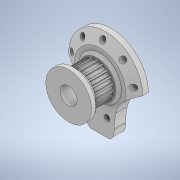
# Autodesk Inventor part: bone_upper_wheel_1
Saved by Autodesk Inventor 2020 (Build 240168000, 168)
## iProperties
Created: 2019-05-05
Part Number: bone_upper_wheel_1
Material: Generic
Document SubType Name: Modeling
Designer: psrob
Density: 1 g/cm^3
Appearance: Default
Author: psrob
Autodesk Inventor part; units mm, degrees
ref_plane "YZ Plane" through (0, 0, 0) normal (1, 0, 0) x (0, 1, 0)
ref_plane "XZ Plane" through (0, 0, 0) normal (0, 1, 0) x (-1, 0, 0)
ref_plane "XY Plane" through (0, 0, 0) normal (0, 0, 1) x (1, 0, 0)
sketch "Sketch1" plane through (0, 0, 0) normal (0, 0, 1) x (1, 0, 0)
  circle A0 centre (0, 18.5) radius 1 projected
  circle A1 centre (7.0707, 15.9265) radius 1 projected
  circle A2 centre (-7.0707, 15.9265) radius 1 projected
  circle A3 centre (10.8329, 9.4101) radius 1 projected
  circle A4 centre (-10.8329, 9.4101) radius 1 projected
  circle A5 centre (0, 7.5) radius 5 projected
  ellipse E0 centre (3, -5.8944) end of major axis (3, -9.5) minor radius 2 (3, -9.5) -> (5, -5.8944) ccw projected
  line L0 (5, -5.8944) -> (5, -5.5) projected
  arc A6 (5.5977, -0.4461) -> (5, -5.5) centre (26.6667, -5.5) ccw projected
  arc A7 (10.155, 5.7831) -> (5.5977, -0.4461) centre (15.3218, -2.7787) ccw projected
  line L1 (10.155, 5.7831) -> (13, 7.5) projected
  arc A8 (13, 7.5) -> (-13, 7.5) centre (0, 7.5) ccw projected
  line L2 (-13, 7.5) -> (-10.155, 5.7831) projected
  arc A9 (-5.5977, -0.4461) -> (-10.155, 5.7831) centre (-15.3218, -2.7787) ccw projected
  arc A10 (-5, -5.5) -> (-5.5977, -0.4461) centre (-26.6667, -5.5) ccw projected
  line L3 (-5, -5.5) -> (-5, -5.8944) projected
  ellipse E1 centre (-3, -5.8944) end of major axis (-3, -9.5) minor radius 2 (-5, -5.8944) -> (-3, -9.5) ccw projected
  line L4 (-3, -9.5) -> (3, -9.5) projected
  circle A11 centre (-2.5, -3.5) radius 1 projected
  circle A12 centre (2.5, -3.5) radius 1 projected
  point P0 (0, 0)
  constraints: 2 other
extrude "Extrusion1" add sketch "Sketch1" along normal blind 4 contours A5 | L4 E1 L3 A10 A9 L2 A8 L1 A7 A6 L0 E0
sketch "Sketch2" plane through (0, 0, 4) normal (0, 0, 1) x (1, 0, 0)
  circle A0 centre (0, 7.5) radius 3 projected
  circle A1 centre (0, 7.5) radius 3
  point P0 (0, 0)
  dimension "d2" = 6
  constraints: 1 centre point, 1 coincident
  measures "d2" diameter of A1
extrude "Extrusion2" cut sketch "Sketch2" against normal blind 3
sketch "Sketch3" plane through (0, 0, 4) normal (0, 0, 1) x (1, 0, 0)
  circle A0 centre (0, 7.5) radius 2.5 projected
  arc A1 (3.5741, 2.5417) -> (3.6111, 2.7467) centre (3.4864, 2.6633) ccw projected
  arc A2 (3.4957, 2.9808) -> (3.6111, 2.7467) centre (4.4426, 3.3021) ccw projected
  arc A3 (4.2392, 3.6696) -> (3.4957, 2.9808) centre (4.0212, 3.1591) ccw projected
  arc A4 (4.4638, 3.5366) -> (4.2392, 3.6696) centre (3.8465, 2.7499) ccw projected
  arc A5 (4.4638, 3.5366) -> (4.671, 3.5579) centre (4.5564, 3.6546) ccw projected
  arc A6 (4.671, 3.5579) -> (4.9313, 3.8888) centre (0, 7.5) ccw projected
  arc A7 (4.9313, 3.8888) -> (4.9032, 4.0952) centre (4.8103, 3.9774) ccw projected
  arc A8 (4.7211, 4.2822) -> (4.9032, 4.0952) centre (5.5224, 4.8804) ccw projected
  arc A9 (5.2154, 5.167) -> (4.7211, 4.2822) centre (5.1658, 4.6142) ccw projected
  arc A10 (5.4701, 5.11) -> (5.2154, 5.167) centre (5.1261, 4.171) ccw projected
  arc A11 (5.4701, 5.11) -> (5.6606, 5.1942) centre (5.5217, 5.2508) ccw projected
  arc A12 (5.6606, 5.1942) -> (5.8059, 5.5894) centre (0, 7.5) ccw projected
  arc A13 (5.8059, 5.5894) -> (5.7154, 5.777) centre (5.6634, 5.6363) ccw projected
  arc A14 (5.4844, 5.8986) -> (5.7154, 5.777) centre (6.0616, 6.7152) ccw projected
  arc A15 (5.681, 6.8928) -> (5.4844, 5.8986) centre (5.8047, 6.3518) ccw projected
  arc A16 (5.9409, 6.9173) -> (5.681, 6.8928) centre (5.9039, 5.918) ccw projected
  arc A17 (5.9409, 6.9173) -> (6.0961, 7.0563) centre (5.9465, 7.0672) ccw projected
  arc A18 (6.0961, 7.0563) -> (6.1122, 7.477) centre (0, 7.5) ccw projected
  arc A19 (6.1122, 7.477) -> (5.9681, 7.6275) centre (5.9622, 7.4776) ccw projected
  arc A20 (5.7108, 7.6717) -> (5.9681, 7.6275) centre (6.0075, 8.6267) ccw projected
  arc A21 (5.5906, 8.6781) -> (5.7108, 7.6717) centre (5.8754, 8.2017) ccw projected
  arc A22 (5.8302, 8.7817) -> (5.5906, 8.6781) centre (6.1038, 7.8198) ccw projected
  arc A23 (5.8302, 8.7817) -> (5.9348, 8.9618) centre (5.7892, 8.9259) ccw projected
  arc A24 (5.9348, 8.9618) -> (5.8201, 9.3669) centre (0, 7.5) ccw projected
  arc A25 (5.8201, 9.3669) -> (5.6366, 9.4655) centre (5.6773, 9.3211) ccw projected
  arc A26 (5.3782, 9.4281) -> (5.6366, 9.4655) centre (5.3653, 10.428) ccw projected
  arc A27 (4.9529, 10.348) -> (5.3782, 9.4281) centre (5.371, 9.983) ccw projected
  arc A28 (5.1488, 10.5206) -> (4.9529, 10.348) centre (5.7063, 9.6904) ccw projected
  arc A29 (5.1488, 10.5206) -> (5.1926, 10.7242) centre (5.0652, 10.6451) ccw projected
  arc A30 (5.1926, 10.7242) -> (4.9583, 11.0741) centre (0, 7.5) ccw projected
  arc A31 (4.9583, 11.0741) -> (4.7533, 11.1111) centre (4.8367, 10.9864) ccw projected
  arc A32 (4.5192, 10.9957) -> (4.7533, 11.1111) centre (4.1979, 11.9426) ccw projected
  arc A33 (3.8304, 11.7392) -> (4.5192, 10.9957) centre (4.3409, 11.5212) ccw projected
  arc A34 (3.9634, 11.9638) -> (3.8304, 11.7392) centre (4.7501, 11.3465) ccw projected
  arc A35 (3.9634, 11.9638) -> (3.9421, 12.171) centre (3.8454, 12.0564) ccw projected
  arc A36 (3.9421, 12.171) -> (3.6112, 12.4313) centre (0, 7.5) ccw projected
  arc A37 (3.6112, 12.4313) -> (3.4048, 12.4032) centre (3.5226, 12.3103) ccw projected
  arc A38 (3.2178, 12.2211) -> (3.4048, 12.4032) centre (2.6196, 13.0224) ccw projected
  arc A39 (2.333, 12.7154) -> (3.2178, 12.2211) centre (2.8858, 12.6658) ccw projected
  arc A40 (2.39, 12.9701) -> (2.333, 12.7154) centre (3.329, 12.6261) ccw projected
  arc A41 (2.39, 12.9701) -> (2.3058, 13.1606) centre (2.2492, 13.0217) ccw projected
  arc A42 (2.3058, 13.1606) -> (1.9106, 13.3059) centre (0, 7.5) ccw projected
  arc A43 (1.9106, 13.3059) -> (1.723, 13.2154) centre (1.8637, 13.1634) ccw projected
  arc A44 (1.6014, 12.9844) -> (1.723, 13.2154) centre (0.7848, 13.5616) ccw projected
  arc A45 (0.6072, 13.181) -> (1.6014, 12.9844) centre (1.1482, 13.3047) ccw projected
  arc A46 (0.5827, 13.4409) -> (0.6072, 13.181) centre (1.582, 13.4039) ccw projected
  arc A47 (0.5827, 13.4409) -> (0.4437, 13.5961) centre (0.4328, 13.4465) ccw projected
  arc A48 (0.4437, 13.5961) -> (0.023, 13.6122) centre (0, 7.5) ccw projected
  arc A49 (0.023, 13.6122) -> (-0.1275, 13.4681) centre (0.0224, 13.4622) ccw projected
  arc A50 (-0.1717, 13.2108) -> (-0.1275, 13.4681) centre (-1.1267, 13.5075) ccw projected
  arc A51 (-1.1781, 13.0906) -> (-0.1717, 13.2108) centre (-0.7017, 13.3754) ccw projected
  arc A52 (-1.2817, 13.3302) -> (-1.1781, 13.0906) centre (-0.3198, 13.6038) ccw projected
  arc A53 (-1.2817, 13.3302) -> (-1.4618, 13.4348) centre (-1.4259, 13.2892) ccw projected
  arc A54 (-1.4618, 13.4348) -> (-1.8669, 13.3201) centre (0, 7.5) ccw projected
  arc A55 (-1.8669, 13.3201) -> (-1.9655, 13.1366) centre (-1.8211, 13.1773) ccw projected
  arc A56 (-1.9281, 12.8782) -> (-1.9655, 13.1366) centre (-2.928, 12.8653) ccw projected
  arc A57 (-2.848, 12.4529) -> (-1.9281, 12.8782) centre (-2.483, 12.871) ccw projected
  arc A58 (-3.0206, 12.6488) -> (-2.848, 12.4529) centre (-2.1904, 13.2063) ccw projected
  arc A59 (-3.0206, 12.6488) -> (-3.2242, 12.6926) centre (-3.1451, 12.5652) ccw projected
  arc A60 (-3.2242, 12.6926) -> (-3.5741, 12.4583) centre (0, 7.5) ccw projected
  arc A61 (-3.5741, 12.4583) -> (-3.6111, 12.2533) centre (-3.4864, 12.3367) ccw projected
  arc A62 (-3.4957, 12.0192) -> (-3.6111, 12.2533) centre (-4.4426, 11.6979) ccw projected
  arc A63 (-4.2392, 11.3304) -> (-3.4957, 12.0192) centre (-4.0212, 11.8409) ccw projected
  arc A64 (-4.4638, 11.4634) -> (-4.2392, 11.3304) centre (-3.8465, 12.2501) ccw projected
  arc A65 (-4.4638, 11.4634) -> (-4.671, 11.4421) centre (-4.5564, 11.3454) ccw projected
  arc A66 (-4.671, 11.4421) -> (-4.9313, 11.1112) centre (0, 7.5) ccw projected
  arc A67 (-4.9313, 11.1112) -> (-4.9032, 10.9048) centre (-4.8103, 11.0226) ccw projected
  arc A68 (-4.7211, 10.7178) -> (-4.9032, 10.9048) centre (-5.5224, 10.1196) ccw projected
  arc A69 (-5.2154, 9.833) -> (-4.7211, 10.7178) centre (-5.1658, 10.3858) ccw projected
  arc A70 (-5.4701, 9.89) -> (-5.2154, 9.833) centre (-5.1261, 10.829) ccw projected
  arc A71 (-5.4701, 9.89) -> (-5.6606, 9.8058) centre (-5.5217, 9.7492) ccw projected
  arc A72 (-5.6606, 9.8058) -> (-5.8059, 9.4106) centre (0, 7.5) ccw projected
  arc A73 (-5.8059, 9.4106) -> (-5.7154, 9.223) centre (-5.6634, 9.3637) ccw projected
  arc A74 (-5.4844, 9.1014) -> (-5.7154, 9.223) centre (-6.0616, 8.2848) ccw projected
  arc A75 (-5.681, 8.1072) -> (-5.4844, 9.1014) centre (-5.8047, 8.6482) ccw projected
  arc A76 (-5.9409, 8.0827) -> (-5.681, 8.1072) centre (-5.9039, 9.082) ccw projected
  arc A77 (-5.9409, 8.0827) -> (-6.0961, 7.9437) centre (-5.9465, 7.9328) ccw projected
  arc A78 (-6.0961, 7.9437) -> (-6.1122, 7.523) centre (0, 7.5) ccw projected
  arc A79 (-6.1122, 7.523) -> (-5.9681, 7.3725) centre (-5.9622, 7.5224) ccw projected
  arc A80 (-5.7108, 7.3283) -> (-5.9681, 7.3725) centre (-6.0075, 6.3733) ccw projected
  arc A81 (-5.5906, 6.3219) -> (-5.7108, 7.3283) centre (-5.8754, 6.7983) ccw projected
  arc A82 (-5.8302, 6.2183) -> (-5.5906, 6.3219) centre (-6.1038, 7.1802) ccw projected
  arc A83 (-5.8302, 6.2183) -> (-5.9348, 6.0382) centre (-5.7892, 6.0741) ccw projected
  arc A84 (-5.9348, 6.0382) -> (-5.8201, 5.6331) centre (0, 7.5) ccw projected
  arc A85 (-5.8201, 5.6331) -> (-5.6366, 5.5345) centre (-5.6773, 5.6789) ccw projected
  arc A86 (-5.3782, 5.5719) -> (-5.6366, 5.5345) centre (-5.3653, 4.572) ccw projected
  arc A87 (-4.9529, 4.652) -> (-5.3782, 5.5719) centre (-5.371, 5.017) ccw projected
  arc A88 (-5.1488, 4.4794) -> (-4.9529, 4.652) centre (-5.7063, 5.3096) ccw projected
  arc A89 (-5.1488, 4.4794) -> (-5.1926, 4.2758) centre (-5.0652, 4.3549) ccw projected
  arc A90 (-5.1926, 4.2758) -> (-4.9583, 3.9259) centre (0, 7.5) ccw projected
  arc A91 (-4.9583, 3.9259) -> (-4.7533, 3.8889) centre (-4.8367, 4.0136) ccw projected
  arc A92 (-4.5192, 4.0043) -> (-4.7533, 3.8889) centre (-4.1979, 3.0574) ccw projected
  arc A93 (-3.8304, 3.2608) -> (-4.5192, 4.0043) centre (-4.3409, 3.4788) ccw projected
  arc A94 (-3.9634, 3.0362) -> (-3.8304, 3.2608) centre (-4.7501, 3.6535) ccw projected
  arc A95 (-3.9634, 3.0362) -> (-3.9421, 2.829) centre (-3.8454, 2.9436) ccw projected
  arc A96 (-3.9421, 2.829) -> (-3.6112, 2.5687) centre (0, 7.5) ccw projected
  arc A97 (-3.6112, 2.5687) -> (-3.4048, 2.5968) centre (-3.5226, 2.6897) ccw projected
  arc A98 (-3.2178, 2.7789) -> (-3.4048, 2.5968) centre (-2.6196, 1.9776) ccw projected
  arc A99 (-2.333, 2.2846) -> (-3.2178, 2.7789) centre (-2.8858, 2.3342) ccw projected
  arc A100 (-2.39, 2.0299) -> (-2.333, 2.2846) centre (-3.329, 2.3739) ccw projected
  arc A101 (-2.39, 2.0299) -> (-2.3058, 1.8394) centre (-2.2492, 1.9783) ccw projected
  arc A102 (-2.3058, 1.8394) -> (-1.9106, 1.6941) centre (0, 7.5) ccw projected
  arc A103 (-1.9106, 1.6941) -> (-1.723, 1.7846) centre (-1.8637, 1.8366) ccw projected
  arc A104 (-1.6014, 2.0156) -> (-1.723, 1.7846) centre (-0.7848, 1.4384) ccw projected
  arc A105 (-0.6072, 1.819) -> (-1.6014, 2.0156) centre (-1.1482, 1.6953) ccw projected
  arc A106 (-0.5827, 1.5591) -> (-0.6072, 1.819) centre (-1.582, 1.5961) ccw projected
  arc A107 (-0.5827, 1.5591) -> (-0.4437, 1.4039) centre (-0.4328, 1.5535) ccw projected
  arc A108 (-0.4437, 1.4039) -> (-0.023, 1.3878) centre (0, 7.5) ccw projected
  arc A109 (-0.023, 1.3878) -> (0.1275, 1.5319) centre (-0.0224, 1.5378) ccw projected
  arc A110 (0.1717, 1.7892) -> (0.1275, 1.5319) centre (1.1267, 1.4925) ccw projected
  arc A111 (1.1781, 1.9094) -> (0.1717, 1.7892) centre (0.7017, 1.6246) ccw projected
  arc A112 (1.2817, 1.6698) -> (1.1781, 1.9094) centre (0.3198, 1.3962) ccw projected
  arc A113 (1.2817, 1.6698) -> (1.4618, 1.5652) centre (1.4259, 1.7108) ccw projected
  arc A114 (1.4618, 1.5652) -> (1.8669, 1.6799) centre (0, 7.5) ccw projected
  arc A115 (1.8669, 1.6799) -> (1.9655, 1.8634) centre (1.8211, 1.8227) ccw projected
  arc A116 (1.9281, 2.1218) -> (1.9655, 1.8634) centre (2.928, 2.1347) ccw projected
  arc A117 (2.848, 2.5471) -> (1.9281, 2.1218) centre (2.483, 2.129) ccw projected
  arc A118 (3.0206, 2.3512) -> (2.848, 2.5471) centre (2.1904, 1.7937) ccw projected
  arc A119 (3.0206, 2.3512) -> (3.2242, 2.3074) centre (3.1451, 2.4348) ccw projected
  arc A120 (3.2242, 2.3074) -> (3.5741, 2.5417) centre (0, 7.5) ccw projected
  circle A121 centre (0, 7.5) radius 3 projected
  point P0 (0, 0)
extrude "Extrusion3" add sketch "Sketch3" along normal blind 8 contours A120 A119 A118 A117 A116 A115 A114 A113 A112 A111 A110 A109 A108 A107 A106 A105 A104 A103 A102 A101 A100 A99 A98 A97 A96 A95 A94 A93 A92 A91 A90 A89 A88 A87 A86 A85 A84 A83 A82 A81 A80 A79 A78 A77 A76 A75 A74 A73 A72 A71 A70 A69 A68 A67 A66 A65 A64 A63 A62 A61 A60 A59 A58 A57 A56 A55 A54 A53 A52 A51 A50 A49 A48 A47 A46 A45 A44 A43 A42 A41 A40 A39 A38 A37 A36 A35 A34 A33 A32 A31 A30 A29 A28 A27 A26 A25 A24 A23 A22 A21 A20 A19 A18 A17 A16 A15 A14 A13 A12 A11 A10 A9 A8 A7 A6 A5 A4 A3 A2 A1
sketch "Sketch4" plane through (0, 0, 4) normal (0, 0, 1) x (1, 0, 0)
  arc A0 (-2.333, 2.2846) -> (-3.2178, 2.7789) centre (-2.8858, 2.3342) ccw projected
  arc A1 (-3.2178, 2.7789) -> (-3.4048, 2.5968) centre (-2.6196, 1.9776) ccw projected
  arc A2 (-3.6112, 2.5687) -> (-3.4048, 2.5968) centre (-3.5226, 2.6897) ccw projected
  arc A3 (-3.9421, 2.829) -> (-3.6112, 2.5687) centre (0, 7.5) ccw projected
  arc A4 (-3.9634, 3.0362) -> (-3.9421, 2.829) centre (-3.8454, 2.9436) ccw projected
  arc A5 (-3.9634, 3.0362) -> (-3.8304, 3.2608) centre (-4.7501, 3.6535) ccw projected
  arc A6 (-3.8304, 3.2608) -> (-4.5192, 4.0043) centre (-4.3409, 3.4788) ccw projected
  arc A7 (-4.5192, 4.0043) -> (-4.7533, 3.8889) centre (-4.1979, 3.0574) ccw projected
  arc A8 (-4.9583, 3.9259) -> (-4.7533, 3.8889) centre (-4.8367, 4.0136) ccw projected
  arc A9 (-5.1926, 4.2758) -> (-4.9583, 3.9259) centre (0, 7.5) ccw projected
  arc A10 (-5.1488, 4.4794) -> (-5.1926, 4.2758) centre (-5.0652, 4.3549) ccw projected
  arc A11 (-5.1488, 4.4794) -> (-4.9529, 4.652) centre (-5.7063, 5.3096) ccw projected
  arc A12 (-4.9529, 4.652) -> (-5.3782, 5.5719) centre (-5.371, 5.017) ccw projected
  arc A13 (-5.3782, 5.5719) -> (-5.6366, 5.5345) centre (-5.3653, 4.572) ccw projected
  arc A14 (-5.8201, 5.6331) -> (-5.6366, 5.5345) centre (-5.6773, 5.6789) ccw projected
  arc A15 (-5.9348, 6.0382) -> (-5.8201, 5.6331) centre (0, 7.5) ccw projected
  arc A16 (-5.8302, 6.2183) -> (-5.9348, 6.0382) centre (-5.7892, 6.0741) ccw projected
  arc A17 (-5.8302, 6.2183) -> (-5.5906, 6.3219) centre (-6.1038, 7.1802) ccw projected
  arc A18 (-5.5906, 6.3219) -> (-5.7108, 7.3283) centre (-5.8754, 6.7983) ccw projected
  arc A19 (-5.7108, 7.3283) -> (-5.9681, 7.3725) centre (-6.0075, 6.3733) ccw projected
  arc A20 (-6.1122, 7.523) -> (-5.9681, 7.3725) centre (-5.9622, 7.5224) ccw projected
  arc A21 (-6.0961, 7.9437) -> (-6.1122, 7.523) centre (0, 7.5) ccw projected
  arc A22 (-5.9409, 8.0827) -> (-6.0961, 7.9437) centre (-5.9465, 7.9328) ccw projected
  arc A23 (-5.9409, 8.0827) -> (-5.681, 8.1072) centre (-5.9039, 9.082) ccw projected
  arc A24 (-5.681, 8.1072) -> (-5.4844, 9.1014) centre (-5.8047, 8.6482) ccw projected
  arc A25 (-5.4844, 9.1014) -> (-5.7154, 9.223) centre (-6.0616, 8.2848) ccw projected
  arc A26 (-5.8059, 9.4106) -> (-5.7154, 9.223) centre (-5.6634, 9.3637) ccw projected
  arc A27 (-5.6606, 9.8058) -> (-5.8059, 9.4106) centre (0, 7.5) ccw projected
  arc A28 (-5.4701, 9.89) -> (-5.6606, 9.8058) centre (-5.5217, 9.7492) ccw projected
  arc A29 (-5.4701, 9.89) -> (-5.2154, 9.833) centre (-5.1261, 10.829) ccw projected
  arc A30 (-5.2154, 9.833) -> (-4.7211, 10.7178) centre (-5.1658, 10.3858) ccw projected
  arc A31 (-4.7211, 10.7178) -> (-4.9032, 10.9048) centre (-5.5224, 10.1196) ccw projected
  arc A32 (-4.9313, 11.1112) -> (-4.9032, 10.9048) centre (-4.8103, 11.0226) ccw projected
  arc A33 (-4.671, 11.4421) -> (-4.9313, 11.1112) centre (0, 7.5) ccw projected
  arc A34 (-4.4638, 11.4634) -> (-4.671, 11.4421) centre (-4.5564, 11.3454) ccw projected
  arc A35 (-4.4638, 11.4634) -> (-4.2392, 11.3304) centre (-3.8465, 12.2501) ccw projected
  arc A36 (-4.2392, 11.3304) -> (-3.4957, 12.0192) centre (-4.0212, 11.8409) ccw projected
  arc A37 (-3.4957, 12.0192) -> (-3.6111, 12.2533) centre (-4.4426, 11.6979) ccw projected
  arc A38 (-3.5741, 12.4583) -> (-3.6111, 12.2533) centre (-3.4864, 12.3367) ccw projected
  arc A39 (-3.2242, 12.6926) -> (-3.5741, 12.4583) centre (0, 7.5) ccw projected
  arc A40 (-3.0206, 12.6488) -> (-3.2242, 12.6926) centre (-3.1451, 12.5652) ccw projected
  arc A41 (-3.0206, 12.6488) -> (-2.848, 12.4529) centre (-2.1904, 13.2063) ccw projected
  arc A42 (-2.848, 12.4529) -> (-1.9281, 12.8782) centre (-2.483, 12.871) ccw projected
  arc A43 (-1.9281, 12.8782) -> (-1.9655, 13.1366) centre (-2.928, 12.8653) ccw projected
  arc A44 (-1.8669, 13.3201) -> (-1.9655, 13.1366) centre (-1.8211, 13.1773) ccw projected
  arc A45 (-1.4618, 13.4348) -> (-1.8669, 13.3201) centre (0, 7.5) ccw projected
  arc A46 (-1.2817, 13.3302) -> (-1.4618, 13.4348) centre (-1.4259, 13.2892) ccw projected
  arc A47 (-1.2817, 13.3302) -> (-1.1781, 13.0906) centre (-0.3198, 13.6038) ccw projected
  arc A48 (-1.1781, 13.0906) -> (-0.1717, 13.2108) centre (-0.7017, 13.3754) ccw projected
  arc A49 (-0.1717, 13.2108) -> (-0.1275, 13.4681) centre (-1.1267, 13.5075) ccw projected
  arc A50 (0.023, 13.6122) -> (-0.1275, 13.4681) centre (0.0224, 13.4622) ccw projected
  arc A51 (0.4437, 13.5961) -> (0.023, 13.6122) centre (0, 7.5) ccw projected
  arc A52 (0.5827, 13.4409) -> (0.4437, 13.5961) centre (0.4328, 13.4465) ccw projected
  arc A53 (0.5827, 13.4409) -> (0.6072, 13.181) centre (1.582, 13.4039) ccw projected
  arc A54 (0.6072, 13.181) -> (1.6014, 12.9844) centre (1.1482, 13.3047) ccw projected
  arc A55 (1.6014, 12.9844) -> (1.723, 13.2154) centre (0.7848, 13.5616) ccw projected
  arc A56 (1.9106, 13.3059) -> (1.723, 13.2154) centre (1.8637, 13.1634) ccw projected
  arc A57 (2.3058, 13.1606) -> (1.9106, 13.3059) centre (0, 7.5) ccw projected
  arc A58 (2.39, 12.9701) -> (2.3058, 13.1606) centre (2.2492, 13.0217) ccw projected
  arc A59 (2.39, 12.9701) -> (2.333, 12.7154) centre (3.329, 12.6261) ccw projected
  arc A60 (2.333, 12.7154) -> (3.2178, 12.2211) centre (2.8858, 12.6658) ccw projected
  arc A61 (3.2178, 12.2211) -> (3.4048, 12.4032) centre (2.6196, 13.0224) ccw projected
  arc A62 (3.6112, 12.4313) -> (3.4048, 12.4032) centre (3.5226, 12.3103) ccw projected
  arc A63 (3.9421, 12.171) -> (3.6112, 12.4313) centre (0, 7.5) ccw projected
  arc A64 (3.9634, 11.9638) -> (3.9421, 12.171) centre (3.8454, 12.0564) ccw projected
  arc A65 (3.9634, 11.9638) -> (3.8304, 11.7392) centre (4.7501, 11.3465) ccw projected
  arc A66 (3.8304, 11.7392) -> (4.5192, 10.9957) centre (4.3409, 11.5212) ccw projected
  arc A67 (4.5192, 10.9957) -> (4.7533, 11.1111) centre (4.1979, 11.9426) ccw projected
  arc A68 (4.9583, 11.0741) -> (4.7533, 11.1111) centre (4.8367, 10.9864) ccw projected
  arc A69 (5.1926, 10.7242) -> (4.9583, 11.0741) centre (0, 7.5) ccw projected
  arc A70 (5.1488, 10.5206) -> (5.1926, 10.7242) centre (5.0652, 10.6451) ccw projected
  arc A71 (5.1488, 10.5206) -> (4.9529, 10.348) centre (5.7063, 9.6904) ccw projected
  arc A72 (4.9529, 10.348) -> (5.3782, 9.4281) centre (5.371, 9.983) ccw projected
  arc A73 (5.3782, 9.4281) -> (5.6366, 9.4655) centre (5.3653, 10.428) ccw projected
  arc A74 (5.8201, 9.3669) -> (5.6366, 9.4655) centre (5.6773, 9.3211) ccw projected
  arc A75 (5.9348, 8.9618) -> (5.8201, 9.3669) centre (0, 7.5) ccw projected
  arc A76 (5.8302, 8.7817) -> (5.9348, 8.9618) centre (5.7892, 8.9259) ccw projected
  arc A77 (5.8302, 8.7817) -> (5.5906, 8.6781) centre (6.1038, 7.8198) ccw projected
  arc A78 (5.5906, 8.6781) -> (5.7108, 7.6717) centre (5.8754, 8.2017) ccw projected
  arc A79 (5.7108, 7.6717) -> (5.9681, 7.6275) centre (6.0075, 8.6267) ccw projected
  arc A80 (6.1122, 7.477) -> (5.9681, 7.6275) centre (5.9622, 7.4776) ccw projected
  arc A81 (6.0961, 7.0563) -> (6.1122, 7.477) centre (0, 7.5) ccw projected
  arc A82 (5.9409, 6.9173) -> (6.0961, 7.0563) centre (5.9465, 7.0672) ccw projected
  arc A83 (5.9409, 6.9173) -> (5.681, 6.8928) centre (5.9039, 5.918) ccw projected
  arc A84 (5.681, 6.8928) -> (5.4844, 5.8986) centre (5.8047, 6.3518) ccw projected
  arc A85 (5.4844, 5.8986) -> (5.7154, 5.777) centre (6.0616, 6.7152) ccw projected
  arc A86 (5.8059, 5.5894) -> (5.7154, 5.777) centre (5.6634, 5.6363) ccw projected
  arc A87 (5.6606, 5.1942) -> (5.8059, 5.5894) centre (0, 7.5) ccw projected
  arc A88 (5.4701, 5.11) -> (5.6606, 5.1942) centre (5.5217, 5.2508) ccw projected
  arc A89 (5.4701, 5.11) -> (5.2154, 5.167) centre (5.1261, 4.171) ccw projected
  arc A90 (5.2154, 5.167) -> (4.7211, 4.2822) centre (5.1658, 4.6142) ccw projected
  arc A91 (4.7211, 4.2822) -> (4.9032, 4.0952) centre (5.5224, 4.8804) ccw projected
  arc A92 (4.9313, 3.8888) -> (4.9032, 4.0952) centre (4.8103, 3.9774) ccw projected
  arc A93 (4.671, 3.5579) -> (4.9313, 3.8888) centre (0, 7.5) ccw projected
  arc A94 (4.4638, 3.5366) -> (4.671, 3.5579) centre (4.5564, 3.6546) ccw projected
  arc A95 (4.4638, 3.5366) -> (4.2392, 3.6696) centre (3.8465, 2.7499) ccw projected
  arc A96 (4.2392, 3.6696) -> (3.4957, 2.9808) centre (4.0212, 3.1591) ccw projected
  arc A97 (3.4957, 2.9808) -> (3.6111, 2.7467) centre (4.4426, 3.3021) ccw projected
  arc A98 (3.5741, 2.5417) -> (3.6111, 2.7467) centre (3.4864, 2.6633) ccw projected
  arc A99 (3.2242, 2.3074) -> (3.5741, 2.5417) centre (0, 7.5) ccw projected
  arc A100 (3.0206, 2.3512) -> (3.2242, 2.3074) centre (3.1451, 2.4348) ccw projected
  arc A101 (3.0206, 2.3512) -> (2.848, 2.5471) centre (2.1904, 1.7937) ccw projected
  arc A102 (2.848, 2.5471) -> (1.9281, 2.1218) centre (2.483, 2.129) ccw projected
  arc A103 (1.9281, 2.1218) -> (1.9655, 1.8634) centre (2.928, 2.1347) ccw projected
  arc A104 (1.8669, 1.6799) -> (1.9655, 1.8634) centre (1.8211, 1.8227) ccw projected
  arc A105 (1.4618, 1.5652) -> (1.8669, 1.6799) centre (0, 7.5) ccw projected
  arc A106 (1.2817, 1.6698) -> (1.4618, 1.5652) centre (1.4259, 1.7108) ccw projected
  arc A107 (1.2817, 1.6698) -> (1.1781, 1.9094) centre (0.3198, 1.3962) ccw projected
  arc A108 (1.1781, 1.9094) -> (0.1717, 1.7892) centre (0.7017, 1.6246) ccw projected
  arc A109 (0.1717, 1.7892) -> (0.1275, 1.5319) centre (1.1267, 1.4925) ccw projected
  arc A110 (-0.023, 1.3878) -> (0.1275, 1.5319) centre (-0.0224, 1.5378) ccw projected
  arc A111 (-0.4437, 1.4039) -> (-0.023, 1.3878) centre (0, 7.5) ccw projected
  arc A112 (-0.5827, 1.5591) -> (-0.4437, 1.4039) centre (-0.4328, 1.5535) ccw projected
  arc A113 (-0.5827, 1.5591) -> (-0.6072, 1.819) centre (-1.582, 1.5961) ccw projected
  arc A114 (-0.6072, 1.819) -> (-1.6014, 2.0156) centre (-1.1482, 1.6953) ccw projected
  arc A115 (-1.6014, 2.0156) -> (-1.723, 1.7846) centre (-0.7848, 1.4384) ccw projected
  arc A116 (-1.9106, 1.6941) -> (-1.723, 1.7846) centre (-1.8637, 1.8366) ccw projected
  arc A117 (-2.3058, 1.8394) -> (-1.9106, 1.6941) centre (0, 7.5) ccw projected
  arc A118 (-2.39, 2.0299) -> (-2.3058, 1.8394) centre (-2.2492, 1.9783) ccw projected
  arc A119 (-2.39, 2.0299) -> (-2.333, 2.2846) centre (-3.329, 2.3739) ccw projected
  arc A120 (5.5977, -0.4461) -> (5, -5.5) centre (26.6667, -5.5) ccw projected
  arc A121 (10.155, 5.7831) -> (5.5977, -0.4461) centre (15.3218, -2.7787) ccw projected
  line L0 (10.155, 5.7831) -> (13, 7.5) projected
  arc A122 (13, 7.5) -> (-13, 7.5) centre (0, 7.5) ccw projected
  line L1 (-13, 7.5) -> (-10.155, 5.7831) projected
  arc A123 (-5.5977, -0.4461) -> (-10.155, 5.7831) centre (-15.3218, -2.7787) ccw projected
  arc A124 (-5, -5.5) -> (-5.5977, -0.4461) centre (-26.6667, -5.5) ccw projected
  line L2 (-5, -5.5) -> (-5, -5.8944) projected
  ellipse E0 centre (-3, -5.8944) end of major axis (-3, -9.5) minor radius 2 (-5, -5.8944) -> (-3, -9.5) ccw projected
  line L3 (-3, -9.5) -> (3, -9.5) projected
  ellipse E1 centre (3, -5.8944) end of major axis (3, -9.5) minor radius 2 (3, -9.5) -> (5, -5.8944) ccw projected
  line L4 (5, -5.8944) -> (5, -5.5) projected
  circle A125 centre (-10.8329, 9.4101) radius 1 projected
  circle A126 centre (10.8329, 9.4101) radius 1 projected
  circle A127 centre (-7.0707, 15.9265) radius 1 projected
  circle A128 centre (7.0707, 15.9265) radius 1 projected
  circle A129 centre (0, 18.5) radius 1 projected
  circle A130 centre (2.5, -3.5) radius 1 projected
  circle A131 centre (-2.5, -3.5) radius 1 projected
  circle A132 centre (0, 7.5) radius 7.5
  point P0 (0, 0)
  dimension "d7" = 15
  constraints: 1 centre point, 1 coincident, 2 other
  measures "d7" diameter of A132
extrude "Extrusion4" add sketch "Sketch4" along normal blind 1 contours A0 A1 A2 A3 A4 A5 A6 A7 A8 A9 A10 A11 A12 A13 A14 A15 A16 A17 A18 A19 A20 A21 A22 A23 A24 A25 A26 A27 A28 A29 A30 A31 A32 A33 A34 A35 A36 A37 A38 A39 A40 A41 A42 A43 A44 A45 A46 A47 A48 A49 A50 A51 A52 A53 A54 A55 A56 A57 A58 A59 A60 A61 A62 A63 A64 A65 A66 A67 A68 A69 A70 A71 A72 A73 A74 A75 A76 A77 A78 A79 A80 A81 A82 A83 A84 A85 A86 A87 A88 A89 A90 A91 A92 A93 A94 A95 A96 A97 A98 A99 A100 A101 A102 A103 A104 A105 A106 A107 A108 A109 A110 A111 A112 A113 A114 A115 A116 A117 A118 A119 | A132
chamfer "Chamfer1" distance 1 angle 45 1 edges at (-7.5, 7.5, 5)
sketch "Sketch5" plane through (0, 0, 12) normal (0, 0, 1) x (1, 0, 0)
  arc A0 (-2.39, 2.0299) -> (-2.333, 2.2846) centre (-3.329, 2.3739) ccw projected
  arc A1 (-2.39, 2.0299) -> (-2.3058, 1.8394) centre (-2.2492, 1.9783) ccw projected
  arc A2 (-2.3058, 1.8394) -> (-1.9106, 1.6941) centre (0, 7.5) ccw projected
  arc A3 (-1.9106, 1.6941) -> (-1.723, 1.7846) centre (-1.8637, 1.8366) ccw projected
  arc A4 (-1.6014, 2.0156) -> (-1.723, 1.7846) centre (-0.7848, 1.4384) ccw projected
  arc A5 (-0.6072, 1.819) -> (-1.6014, 2.0156) centre (-1.1482, 1.6953) ccw projected
  arc A6 (-0.5827, 1.5591) -> (-0.6072, 1.819) centre (-1.582, 1.5961) ccw projected
  arc A7 (-0.5827, 1.5591) -> (-0.4437, 1.4039) centre (-0.4328, 1.5535) ccw projected
  arc A8 (-0.4437, 1.4039) -> (-0.023, 1.3878) centre (0, 7.5) ccw projected
  arc A9 (-0.023, 1.3878) -> (0.1275, 1.5319) centre (-0.0224, 1.5378) ccw projected
  arc A10 (0.1717, 1.7892) -> (0.1275, 1.5319) centre (1.1267, 1.4925) ccw projected
  arc A11 (1.1781, 1.9094) -> (0.1717, 1.7892) centre (0.7017, 1.6246) ccw projected
  arc A12 (1.2817, 1.6698) -> (1.1781, 1.9094) centre (0.3198, 1.3962) ccw projected
  arc A13 (1.2817, 1.6698) -> (1.4618, 1.5652) centre (1.4259, 1.7108) ccw projected
  arc A14 (1.4618, 1.5652) -> (1.8669, 1.6799) centre (0, 7.5) ccw projected
  arc A15 (1.8669, 1.6799) -> (1.9655, 1.8634) centre (1.8211, 1.8227) ccw projected
  arc A16 (1.9281, 2.1218) -> (1.9655, 1.8634) centre (2.928, 2.1347) ccw projected
  arc A17 (2.848, 2.5471) -> (1.9281, 2.1218) centre (2.483, 2.129) ccw projected
  arc A18 (3.0206, 2.3512) -> (2.848, 2.5471) centre (2.1904, 1.7937) ccw projected
  arc A19 (3.0206, 2.3512) -> (3.2242, 2.3074) centre (3.1451, 2.4348) ccw projected
  arc A20 (3.2242, 2.3074) -> (3.5741, 2.5417) centre (0, 7.5) ccw projected
  arc A21 (3.5741, 2.5417) -> (3.6111, 2.7467) centre (3.4864, 2.6633) ccw projected
  arc A22 (3.4957, 2.9808) -> (3.6111, 2.7467) centre (4.4426, 3.3021) ccw projected
  arc A23 (4.2392, 3.6696) -> (3.4957, 2.9808) centre (4.0212, 3.1591) ccw projected
  arc A24 (4.4638, 3.5366) -> (4.2392, 3.6696) centre (3.8465, 2.7499) ccw projected
  arc A25 (4.4638, 3.5366) -> (4.671, 3.5579) centre (4.5564, 3.6546) ccw projected
  arc A26 (4.671, 3.5579) -> (4.9313, 3.8888) centre (0, 7.5) ccw projected
  arc A27 (4.9313, 3.8888) -> (4.9032, 4.0952) centre (4.8103, 3.9774) ccw projected
  arc A28 (4.7211, 4.2822) -> (4.9032, 4.0952) centre (5.5224, 4.8804) ccw projected
  arc A29 (5.2154, 5.167) -> (4.7211, 4.2822) centre (5.1658, 4.6142) ccw projected
  arc A30 (5.4701, 5.11) -> (5.2154, 5.167) centre (5.1261, 4.171) ccw projected
  arc A31 (5.4701, 5.11) -> (5.6606, 5.1942) centre (5.5217, 5.2508) ccw projected
  arc A32 (5.6606, 5.1942) -> (5.8059, 5.5894) centre (0, 7.5) ccw projected
  arc A33 (5.8059, 5.5894) -> (5.7154, 5.777) centre (5.6634, 5.6363) ccw projected
  arc A34 (5.4844, 5.8986) -> (5.7154, 5.777) centre (6.0616, 6.7152) ccw projected
  arc A35 (5.681, 6.8928) -> (5.4844, 5.8986) centre (5.8047, 6.3518) ccw projected
  arc A36 (5.9409, 6.9173) -> (5.681, 6.8928) centre (5.9039, 5.918) ccw projected
  arc A37 (5.9409, 6.9173) -> (6.0961, 7.0563) centre (5.9465, 7.0672) ccw projected
  arc A38 (6.0961, 7.0563) -> (6.1122, 7.477) centre (0, 7.5) ccw projected
  arc A39 (6.1122, 7.477) -> (5.9681, 7.6275) centre (5.9622, 7.4776) ccw projected
  arc A40 (5.7108, 7.6717) -> (5.9681, 7.6275) centre (6.0075, 8.6267) ccw projected
  arc A41 (5.5906, 8.6781) -> (5.7108, 7.6717) centre (5.8754, 8.2017) ccw projected
  arc A42 (5.8302, 8.7817) -> (5.5906, 8.6781) centre (6.1038, 7.8198) ccw projected
  arc A43 (5.8302, 8.7817) -> (5.9348, 8.9618) centre (5.7892, 8.9259) ccw projected
  arc A44 (5.9348, 8.9618) -> (5.8201, 9.3669) centre (0, 7.5) ccw projected
  arc A45 (5.8201, 9.3669) -> (5.6366, 9.4655) centre (5.6773, 9.3211) ccw projected
  arc A46 (5.3782, 9.4281) -> (5.6366, 9.4655) centre (5.3653, 10.428) ccw projected
  arc A47 (4.9529, 10.348) -> (5.3782, 9.4281) centre (5.371, 9.983) ccw projected
  arc A48 (5.1488, 10.5206) -> (4.9529, 10.348) centre (5.7063, 9.6904) ccw projected
  arc A49 (5.1488, 10.5206) -> (5.1926, 10.7242) centre (5.0652, 10.6451) ccw projected
  arc A50 (5.1926, 10.7242) -> (4.9583, 11.0741) centre (0, 7.5) ccw projected
  arc A51 (4.9583, 11.0741) -> (4.7533, 11.1111) centre (4.8367, 10.9864) ccw projected
  arc A52 (4.5192, 10.9957) -> (4.7533, 11.1111) centre (4.1979, 11.9426) ccw projected
  arc A53 (3.8304, 11.7392) -> (4.5192, 10.9957) centre (4.3409, 11.5212) ccw projected
  arc A54 (3.9634, 11.9638) -> (3.8304, 11.7392) centre (4.7501, 11.3465) ccw projected
  arc A55 (3.9634, 11.9638) -> (3.9421, 12.171) centre (3.8454, 12.0564) ccw projected
  arc A56 (3.9421, 12.171) -> (3.6112, 12.4313) centre (0, 7.5) ccw projected
  arc A57 (3.6112, 12.4313) -> (3.4048, 12.4032) centre (3.5226, 12.3103) ccw projected
  arc A58 (3.2178, 12.2211) -> (3.4048, 12.4032) centre (2.6196, 13.0224) ccw projected
  arc A59 (2.333, 12.7154) -> (3.2178, 12.2211) centre (2.8858, 12.6658) ccw projected
  arc A60 (2.39, 12.9701) -> (2.333, 12.7154) centre (3.329, 12.6261) ccw projected
  arc A61 (2.39, 12.9701) -> (2.3058, 13.1606) centre (2.2492, 13.0217) ccw projected
  arc A62 (2.3058, 13.1606) -> (1.9106, 13.3059) centre (0, 7.5) ccw projected
  arc A63 (1.9106, 13.3059) -> (1.723, 13.2154) centre (1.8637, 13.1634) ccw projected
  arc A64 (1.6014, 12.9844) -> (1.723, 13.2154) centre (0.7848, 13.5616) ccw projected
  arc A65 (0.6072, 13.181) -> (1.6014, 12.9844) centre (1.1482, 13.3047) ccw projected
  arc A66 (0.5827, 13.4409) -> (0.6072, 13.181) centre (1.582, 13.4039) ccw projected
  arc A67 (0.5827, 13.4409) -> (0.4437, 13.5961) centre (0.4328, 13.4465) ccw projected
  arc A68 (0.4437, 13.5961) -> (0.023, 13.6122) centre (0, 7.5) ccw projected
  arc A69 (0.023, 13.6122) -> (-0.1275, 13.4681) centre (0.0224, 13.4622) ccw projected
  arc A70 (-0.1717, 13.2108) -> (-0.1275, 13.4681) centre (-1.1267, 13.5075) ccw projected
  arc A71 (-1.1781, 13.0906) -> (-0.1717, 13.2108) centre (-0.7017, 13.3754) ccw projected
  arc A72 (-1.2817, 13.3302) -> (-1.1781, 13.0906) centre (-0.3198, 13.6038) ccw projected
  arc A73 (-1.2817, 13.3302) -> (-1.4618, 13.4348) centre (-1.4259, 13.2892) ccw projected
  arc A74 (-1.4618, 13.4348) -> (-1.8669, 13.3201) centre (0, 7.5) ccw projected
  arc A75 (-1.8669, 13.3201) -> (-1.9655, 13.1366) centre (-1.8211, 13.1773) ccw projected
  arc A76 (-1.9281, 12.8782) -> (-1.9655, 13.1366) centre (-2.928, 12.8653) ccw projected
  arc A77 (-2.848, 12.4529) -> (-1.9281, 12.8782) centre (-2.483, 12.871) ccw projected
  arc A78 (-3.0206, 12.6488) -> (-2.848, 12.4529) centre (-2.1904, 13.2063) ccw projected
  arc A79 (-3.0206, 12.6488) -> (-3.2242, 12.6926) centre (-3.1451, 12.5652) ccw projected
  arc A80 (-3.2242, 12.6926) -> (-3.5741, 12.4583) centre (0, 7.5) ccw projected
  arc A81 (-3.5741, 12.4583) -> (-3.6111, 12.2533) centre (-3.4864, 12.3367) ccw projected
  arc A82 (-3.4957, 12.0192) -> (-3.6111, 12.2533) centre (-4.4426, 11.6979) ccw projected
  arc A83 (-4.2392, 11.3304) -> (-3.4957, 12.0192) centre (-4.0212, 11.8409) ccw projected
  arc A84 (-4.4638, 11.4634) -> (-4.2392, 11.3304) centre (-3.8465, 12.2501) ccw projected
  arc A85 (-4.4638, 11.4634) -> (-4.671, 11.4421) centre (-4.5564, 11.3454) ccw projected
  arc A86 (-4.671, 11.4421) -> (-4.9313, 11.1112) centre (0, 7.5) ccw projected
  arc A87 (-4.9313, 11.1112) -> (-4.9032, 10.9048) centre (-4.8103, 11.0226) ccw projected
  arc A88 (-4.7211, 10.7178) -> (-4.9032, 10.9048) centre (-5.5224, 10.1196) ccw projected
  arc A89 (-5.2154, 9.833) -> (-4.7211, 10.7178) centre (-5.1658, 10.3858) ccw projected
  arc A90 (-5.4701, 9.89) -> (-5.2154, 9.833) centre (-5.1261, 10.829) ccw projected
  arc A91 (-5.4701, 9.89) -> (-5.6606, 9.8058) centre (-5.5217, 9.7492) ccw projected
  arc A92 (-5.6606, 9.8058) -> (-5.8059, 9.4106) centre (0, 7.5) ccw projected
  arc A93 (-5.8059, 9.4106) -> (-5.7154, 9.223) centre (-5.6634, 9.3637) ccw projected
  arc A94 (-5.4844, 9.1014) -> (-5.7154, 9.223) centre (-6.0616, 8.2848) ccw projected
  arc A95 (-5.681, 8.1072) -> (-5.4844, 9.1014) centre (-5.8047, 8.6482) ccw projected
  arc A96 (-5.9409, 8.0827) -> (-5.681, 8.1072) centre (-5.9039, 9.082) ccw projected
  arc A97 (-5.9409, 8.0827) -> (-6.0961, 7.9437) centre (-5.9465, 7.9328) ccw projected
  arc A98 (-6.0961, 7.9437) -> (-6.1122, 7.523) centre (0, 7.5) ccw projected
  arc A99 (-6.1122, 7.523) -> (-5.9681, 7.3725) centre (-5.9622, 7.5224) ccw projected
  arc A100 (-5.7108, 7.3283) -> (-5.9681, 7.3725) centre (-6.0075, 6.3733) ccw projected
  arc A101 (-5.5906, 6.3219) -> (-5.7108, 7.3283) centre (-5.8754, 6.7983) ccw projected
  arc A102 (-5.8302, 6.2183) -> (-5.5906, 6.3219) centre (-6.1038, 7.1802) ccw projected
  arc A103 (-5.8302, 6.2183) -> (-5.9348, 6.0382) centre (-5.7892, 6.0741) ccw projected
  arc A104 (-5.9348, 6.0382) -> (-5.8201, 5.6331) centre (0, 7.5) ccw projected
  arc A105 (-5.8201, 5.6331) -> (-5.6366, 5.5345) centre (-5.6773, 5.6789) ccw projected
  arc A106 (-5.3782, 5.5719) -> (-5.6366, 5.5345) centre (-5.3653, 4.572) ccw projected
  arc A107 (-4.9529, 4.652) -> (-5.3782, 5.5719) centre (-5.371, 5.017) ccw projected
  arc A108 (-5.1488, 4.4794) -> (-4.9529, 4.652) centre (-5.7063, 5.3096) ccw projected
  arc A109 (-5.1488, 4.4794) -> (-5.1926, 4.2758) centre (-5.0652, 4.3549) ccw projected
  arc A110 (-5.1926, 4.2758) -> (-4.9583, 3.9259) centre (0, 7.5) ccw projected
  arc A111 (-4.9583, 3.9259) -> (-4.7533, 3.8889) centre (-4.8367, 4.0136) ccw projected
  arc A112 (-4.5192, 4.0043) -> (-4.7533, 3.8889) centre (-4.1979, 3.0574) ccw projected
  arc A113 (-3.8304, 3.2608) -> (-4.5192, 4.0043) centre (-4.3409, 3.4788) ccw projected
  arc A114 (-3.9634, 3.0362) -> (-3.8304, 3.2608) centre (-4.7501, 3.6535) ccw projected
  arc A115 (-3.9634, 3.0362) -> (-3.9421, 2.829) centre (-3.8454, 2.9436) ccw projected
  arc A116 (-3.9421, 2.829) -> (-3.6112, 2.5687) centre (0, 7.5) ccw projected
  arc A117 (-3.6112, 2.5687) -> (-3.4048, 2.5968) centre (-3.5226, 2.6897) ccw projected
  arc A118 (-3.2178, 2.7789) -> (-3.4048, 2.5968) centre (-2.6196, 1.9776) ccw projected
  arc A119 (-2.333, 2.2846) -> (-3.2178, 2.7789) centre (-2.8858, 2.3342) ccw projected
  circle A120 centre (0, 7.5) radius 3 projected
  circle A121 centre (0, 7.5) radius 8
  point P0 (0, 0)
  dimension "d13" = 16
  constraints: 1 centre point, 1 coincident
  measures "d13" diameter of A121
extrude "Extrusion5" add sketch "Sketch5" along normal blind 3 contours A0 A119 A118 A117 A116 A115 A114 A113 A112 A111 A110 A109 A108 A107 A106 A105 A104 A103 A102 A101 A100 A99 A98 A97 A96 A95 A94 A93 A92 A91 A90 A89 A88 A87 A86 A85 A84 A83 A82 A81 A80 A79 A78 A77 A76 A75 A74 A73 A72 A71 A70 A69 A68 A67 A66 A65 A64 A63 A62 A61 A60 A59 A58 A57 A56 A55 A54 A53 A52 A51 A50 A49 A48 A47 A46 A45 A44 A43 A42 A41 A40 A39 A38 A37 A36 A35 A34 A33 A32 A31 A30 A29 A28 A27 A26 A25 A24 A23 A22 A21 A20 A19 A18 A17 A16 A15 A14 A13 A12 A11 A10 A9 A8 A7 A6 A5 A4 A3 A2 A1 | A121
chamfer "Chamfer2" distance 1.5 angle 45 1 edges at (-8, 7.5, 12)
sketch "Sketch6" plane through (0, 0, 0) normal (0, 0, -1) x (-1, 0, 0)
  circle A0 centre (0, 7.5) radius 3 projected
  circle A1 centre (0, 7.5) radius 3
  point P0 (0, 0)
  dimension "d19" = 6
  constraints: 1 centre point, 1 coincident
  measures "d19" diameter of A1
extrude "Extrusion6" cut sketch "Sketch6" against normal blind 20
chamfer "Chamfer3" distance 4 distance2 2 1 edges at (0, 20.5, 4) measured on face at (0, 20, 4)
body "Solid1"
